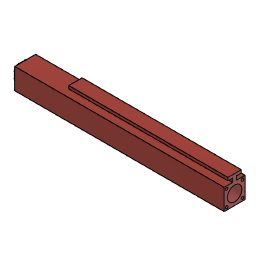
EM2022 Inženýr-ploter (Autodesk Fusion 360 archive; units mm, degrees)
design "EM_22_Plotter_arm_fixa_holder_v7"
Autodesk Fusion 360 part; units mm, degrees
sketch "Sketch7" plane through (0, 0, 0) normal (0, 1, 0) x (1, 0, 0)
sketch "Sketch8" plane through (0, 0, 0) normal (1, 0, 0) x (0, 1, 0)
  circle A0 centre (0, 0) radius 4.6
  line L0 (0, 0) -> (6.5079, 0)
  line L1 (0, 0) -> (0, 4.6)
  line L2 (0, 4.6) -> (0, 6.6)
  line L3 (0, 6.6) -> (6.5777, 6.6)
  line L4 (0, 0) -> (-4.6, 0)
  line L5 (-4.6, 0) -> (-6.6, 0)
  line L6 (0, 0) -> (0, -4.6)
  line L7 (0, -4.6) -> (0, -6.6)
  line L8 (0, -6.6) -> (-6.5261, -6.6)
  line L9 (6.5777, 6.6) -> (-6.5261, 6.6)
  line L10 (-6.5261, -6.6) -> (6.5079, -6.6)
  line L11 (4.6, 0) -> (6.6, 0)
  line L12 (6.6, 0) -> (6.5777, 6.6)
  line L13 (6.5079, 0) -> (6.5079, -6.6)
  line L14 (-6.6, 0) -> (-6.6, -6.5001)
  line L15 (-6.6, 0) -> (-6.6, 6.5001)
  line L16 (0, -6.6) -> (-6.6, -6.6)
  line L17 (-6.6, -6.6) -> (-6.6, -6.4)
  line L18 (-6.5261, 6.6) -> (-6.6, 6.6)
  line L19 (-6.6, 6.6) -> (-6.6, 6.4)
  dimension "d1" = 9.2
  dimension "d2" = 2
  dimension "d3" = 2
  dimension "d4" = 2
  dimension "d5" = 2
  constraint coincident A0.centre L0.start
  constraint horizontal L0
  constraint coincident A0 L1.end
  constraint perpendicular L0 L1
  constraint parallel L1 L2
  constraint perpendicular L2 L3
  constraint coincident A0 L4.end
  constraint perpendicular L1 L4
  constraint parallel L4 L5
  constraint coincident A0 L6.end
  constraint perpendicular L0 L6
  constraint perpendicular L0 L7
  constraint perpendicular L7 L8
  constraint horizontal L9
  constraint horizontal L10
  constraint coincident L0 L11.start
  constraint coincident A0 L11.start
  constraint parallel L0 L11
  constraint perpendicular L10 L13
  constraint vertical L14
  constraint vertical L15
  constraint perpendicular L14 L16
  constraint coincident L14 L17.end
  constraint perpendicular L16 L17
  constraint perpendicular L15 L18
  constraint coincident L15 L19.end
  constraint perpendicular L18 L19
  measures "d1" diameter of A0
  measures "d2" distance of L1.end L2.end
  measures "d3" distance of L4.end L5.end
  measures "d4" distance of L6.end L7.end
  measures "d5" distance of L11.start L11.end
extrude "Extrude1" add sketch "Sketch8" along normal blind 130 contours A0 L0 L7 L10 L11 L13 | A0 L0 L2 L3 L9 L11 L12 | A0 L2 L5 L9 L15 L18 L19 | A0 L5 L7 L8 L10 L14 L16 L17 makes body 1
extrude "Extrude2" add 1 faces at (86.6667, 6.5079, -2.2) along direction (0, 1, 0) blind 0.104 on bodies 1 bodies 1
sketch "Sketch9" plane through (0, 0, 0) normal (-1, 0, 0) x (0, -1, 0)
  circle A0 centre (0, 0) radius 4.6
  line L0 (-6.6, 0) -> (-6.6119, 0)
  line L1 (-6.6119, 0) -> (-6.6119, -6.6)
  line L2 (-6.6119, -6.6) -> (6.6, -6.6)
  line L3 (6.6, -6.6) -> (6.6, 6.6)
  line L4 (6.6, 6.6) -> (-6.5777, 6.6)
  line L5 (-6.5777, 6.6) -> (-6.6, 0)
  circle A1 centre (0, 0) radius 2.75
  line L6 (5, 5) -> (-5, 5)
  line L7 (-5, 5) -> (-5, -5)
  line L8 (-5, -5) -> (5, -5)
  line L9 (5, -5) -> (5, 5)
  dimension "d10" = 5.5
  constraint coincident A0.centre A1.centre
  constraint horizontal L6
  constraint vertical L7
  constraint horizontal L8
  constraint vertical L9
  measures "d10" diameter of A1
extrude "Extrude3" add sketch "Sketch9" along normal blind 4 and the other way blind 0 draft 5 contours A0 | L6 L7 L8 L9 bodies 1
extrude "Extrude4" add 1 faces at (0, 5.5333, 0) along direction (-1, 0, 0) blind 2 on bodies 1 bodies 1
fillet "Fillet1" radius 3 4 edges at (-3, -5, -5) (-3, 5, -5) (-3, -5, 5) (-3, 5, 5) on bodies 1
extrude "Extrude5" cut 1 faces at (42, 6.6119, -4.4) along direction (0, -1, 0) blind 0.002 on bodies 1 bodies 1
fillet "Fillet2" radius 0.6 8 edges at (-4, 4.1213, -4.1213) (-4, 0, -5) (-4, -4.1213, -4.1213) (-4, -5, 0) (-4, -4.1213, 4.1213) (-4, 0, 5) (-4, 4.1213, 4.1213) (-4, 5, 0) on bodies 1
fillet "Fillet3" radius 0.4 8 edges at (-2, -5, 0) (-2, -4.1213, 4.1213) (-2, 0, 5) (-2, 4.1213, 4.1213) (-2, 5, 0) (-2, 4.1213, -4.1213) (-2, 0, -5) (-2, -4.1213, -4.1213) on bodies 1
fillet "Fillet4" radius 0.4 3 edges at (-2, -6.6, 0) (-2, -0.0112, 6.6) (-2, 0.005, -6.6) on bodies 1
sketch "Sketch10" plane through (130, 0, 0) normal (1, 0, 0) x (0, 1, 0)
  line L0 (6.6099, -6.6) -> (6.6099, 0)
  line L1 (6.6099, 0) -> (6.6, 0)
  line L2 (6.6, 0) -> (6.5777, 6.6)
  line L3 (6.5777, 6.6) -> (-6.6, 6.6)
  line L4 (-6.6, 6.6) -> (-6.6, -6.6)
  line L5 (-6.6, -6.6) -> (6.6099, -6.6)
  circle A0 centre (0, 0) radius 4.6
extrude "Extrude6" add sketch "Sketch10" along normal blind 28 separate body makes body 2
sketch "Sketch11" plane through (158, 0, 0) normal (1, 0, 0) x (0, 1, 0)
  circle A0 centre (0, 0) radius 4.6
  line L0 (-6.6, -6.6) -> (6.6099, -6.6)
  line L1 (6.6099, -6.6) -> (6.6099, 0)
  line L2 (6.6099, 0) -> (6.6, 0)
  line L3 (6.6, 0) -> (6.5777, 6.6)
  line L4 (6.5777, 6.6) -> (-6.6, 6.6)
  line L5 (-6.6, 6.6) -> (-6.6, -6.6)
  line L6 (5, 5) -> (-5, 5)
  line L7 (-5, 5) -> (-5, -5)
  line L8 (-5, -5) -> (5, -5)
  line L9 (5, -5) -> (5, 5)
  constraint horizontal L6
  constraint vertical L7
  constraint horizontal L8
  constraint vertical L9
extrude "Extrude7" add sketch "Sketch11" along normal blind 2 and the other way blind 1.5 contours A0 | L6 L7 L8 L9 bodies 2
sketch "Sketch12" plane through (156.5, 0, 0) normal (-1, 0, 0) x (0, -1, 0)
  circle A0 centre (0, 0) radius 4.6
  circle A1 centre (0, 0) radius 2.5
  dimension "d33" = 5
  constraint coincident A0.centre A1.centre
  measures "d33" diameter of A1
extrude "Extrude8" add sketch "Sketch12" along normal blind 26.5 bodies 2
sketch "Sketch13" plane through (130, 0, 0) normal (-1, 0, 0) x (0, -1, 0)
  circle A0 centre (0, 0) radius 2.5
  line L0 (-6.6099, -6.6) -> (6.6, -6.6)
  line L1 (6.6, -6.6) -> (6.6, 6.6)
  line L2 (6.6, 6.6) -> (-6.5777, 6.6)
  line L3 (-6.5777, 6.6) -> (-6.6, 0)
  line L4 (-6.6, 0) -> (-6.6099, 0)
  line L5 (-6.6099, 0) -> (-6.6099, -6.6)
  line L6 (-4, -4) -> (4, -4)
  line L7 (4, -4) -> (4, 4)
  line L8 (4, 4) -> (-4, 4)
  line L9 (-4, 4) -> (-4, -4)
  constraint horizontal L6
  constraint vertical L7
  constraint horizontal L8
  constraint vertical L9
extrude "Extrude9" cut sketch "Sketch13" against normal blind 34 contours L0 L1 L2 L3 L4 L5 bodies 2
sketch "Sketch14" plane through (160, 0, 0) normal (1, 0, 0) x (0, 1, 0)
  line L0 (4, 4) -> (-4, 4)
  line L1 (-4, 4) -> (-4, -4)
  line L2 (-4, -4) -> (4, -4)
  line L3 (4, -4) -> (4, 4)
  line L4 (3, 3) -> (-3, 3)
  line L5 (-3, 3) -> (-3, -3)
  line L6 (-3, -3) -> (3, -3)
  line L7 (3, -3) -> (3, 3)
  constraint horizontal L4
  constraint vertical L5
  constraint horizontal L6
  constraint vertical L7
extrude "Extrude10" add sketch "Sketch14" along normal blind 1 contours L4 L5 L6 L7 bodies 2
sketch "Sketch15" plane through (130, 0, 0) normal (-1, 0, 0) x (0, -1, 0)
  line L0 (4, 4) -> (-4, 4)
  line L1 (-4, 4) -> (-4, -4)
  line L2 (-4, -4) -> (4, -4)
  line L3 (4, -4) -> (4, 4)
  circle A0 centre (0, 0) radius 2.5
  line L4 (5, 5) -> (-5, 5)
  line L5 (-5, 5) -> (-5, -5)
  line L6 (-5, -5) -> (5, -5)
  line L7 (5, -5) -> (5, 5)
  constraint horizontal L4
  constraint vertical L5
  constraint horizontal L6
  constraint vertical L7
extrude "Extrude11" add sketch "Sketch15" against normal blind 30 contours L4 L5 L6 L7 bodies 2
sketch "Sketch16" plane through (130, 0, 0) normal (1, 0, 0) x (0, 1, 0)
  line L0 (6.6099, -6.6) -> (6.6099, 0)
  line L1 (6.6099, 0) -> (6.6, 0)
  line L2 (6.6, 0) -> (6.5777, 6.6)
  line L3 (6.5777, 6.6) -> (-6.6, 6.6)
  line L4 (-6.6, 6.6) -> (-6.6, -6.6)
  line L5 (-6.6, -6.6) -> (6.6099, -6.6)
  circle A0 centre (0, 0) radius 4.6
  circle A1 centre (5, 5) radius 0.85
  circle A2 centre (-5, 5) radius 0.85
  circle A3 centre (5, -5) radius 0.85
  circle A4 centre (-5, -5) radius 0.85
  dimension "d42" = 1.7
  dimension "d43" = 1.7
  dimension "d44" = 1.7
  dimension "d45" = 1.7
  measures "d42" diameter of A1
  measures "d43" diameter of A2
  measures "d44" diameter of A3
  measures "d45" diameter of A4
extrude "Extrude12" cut sketch "Sketch16" against normal blind 7 contours A1 | A2 | A3 | A4 bodies 1
sketch "Sketch17" plane through (160, 0, 0) normal (1, 0, 0) x (0, 1, 0)
  line L0 (-5, 5) -> (-5, -5)
  line L1 (-5, -5) -> (5, -5)
  line L2 (5, -5) -> (5, 5)
  line L3 (5, 5) -> (-5, 5)
  line L4 (3, -3) -> (-3, -3)
  line L5 (-3, -3) -> (-3, 3)
  line L6 (-3, 3) -> (3, 3)
  line L7 (3, 3) -> (3, -3)
  circle A0 centre (5, 5) radius 0.85
  circle A1 centre (-5, 5) radius 0.85
  circle A2 centre (-5, -5) radius 0.85
  circle A3 centre (5, -5) radius 0.85
  circle A4 centre (5, -5) radius 1.6
  circle A5 centre (5, 5) radius 1.6
  circle A6 centre (-5, 5) radius 1.6
  circle A7 centre (-5, -5) radius 1.6
  dimension "d48" = 1.7
  dimension "d49" = 1.7
  dimension "d50" = 1.7
  dimension "d51" = 1.7
  constraint coincident L2.end L3.start
  constraint coincident L0.start L3.end
  constraint coincident L0.end L1.start
  constraint coincident L1.end L2.start
  constraint concentric A3 A4
  constraint concentric A1 A6
  constraint concentric A2 A7
  measures "d48" diameter of A0
  measures "d49" diameter of A1
  measures "d50" diameter of A2
  measures "d51" diameter of A3
extrude "Extrude13" add sketch "Sketch17" along normal blind -30 and the other way blind 27 contours L0 L3 A1 A6 | L0 L1 A2 A7 | L2 L3 A0 A5 | L1 L2 A3 A4 picked at (-6.3454, 4.9461) picked at (-3.6588, -5.1198) picked at (3.9607, 5.8559) picked at (3.656, -5.0795) bodies 2
sketch "Sketch18" plane through (0, 0, 0) normal (0, 0, 1) x (1, 0, 0)
sketch "Sketch19" plane through (130, 0, 0) normal (-1, 0, 0) x (0, -1, 0)
  line L0 (-4.15, 5) -> (-5, 5)
  line L1 (-5, 5) -> (-5, 4.15)
  arc A0 (-4.15, 5) -> (-5, 4.15) centre (-5, 5) ccw
  arc A1 (-3.4, 5) -> (-5, 3.4) centre (-5, 5) ccw
  line L2 (-5, 3.4) -> (-5, -3.4)
  arc A2 (-5, -3.4) -> (-3.4, -5) centre (-5, -5) ccw
  line L3 (-3.4, -5) -> (3.4, -5)
  arc A3 (3.4, -5) -> (5, -3.4) centre (5, -5) ccw
  line L4 (5, -3.4) -> (5, 3.4)
  arc A4 (5, 3.4) -> (3.4, 5) centre (5, 5) ccw
  line L5 (3.4, 5) -> (-3.4, 5)
  line L6 (-5, -4.15) -> (-5, -5)
  line L7 (-5, -5) -> (-4.15, -5)
  arc A5 (-5, -4.15) -> (-4.15, -5) centre (-5, -5) ccw
  arc A6 (4.15, -5) -> (5, -4.15) centre (5, -5) ccw
  line L8 (4.15, -5) -> (5, -5)
  line L9 (5, -5) -> (5, -4.15)
  arc A7 (5, 4.15) -> (4.15, 5) centre (5, 5) ccw
  line L10 (5, 4.15) -> (5, 5)
  line L11 (5, 5) -> (4.15, 5)
  circle A8 centre (0, 0) radius 2.5
  circle A9 centre (-5, 5) radius 0.85
  circle A10 centre (-5, -5) radius 0.85
  circle A11 centre (5, 5) radius 0.85
  circle A12 centre (5, -5) radius 0.85
  constraint coincident L1.end A9
  constraint concentric A2 A10
  constraint coincident L6.start A10
  constraint concentric A4 A11
  constraint concentric A3 A12
extrude "Extrude14" cut sketch "Sketch19" against normal blind 34 contours L0 L1 A9 | L6 L7 A10 | L8 L9 A12 | L10 L11 A11 bodies 2
sketch "Sketch20" plane through (160, 0, 0) normal (1, 0, 0) x (0, 1, 0)
  line L0 (3, -3) -> (-3, -3)
  line L1 (-3, -3) -> (-3, 3)
  line L2 (-3, 3) -> (3, 3)
  line L3 (3, 3) -> (3, -3)
  arc A0 (-5, 4.15) -> (-4.15, 5) centre (-5, 5) ccw
  line L4 (-5, 4.15) -> (-5, -4.15)
  arc A1 (-4.15, -5) -> (-5, -4.15) centre (-5, -5) ccw
  line L5 (-4.15, -5) -> (4.15, -5)
  arc A2 (5, -4.15) -> (4.15, -5) centre (5, -5) ccw
  line L6 (5, -4.15) -> (5, 4.15)
  arc A3 (4.15, 5) -> (5, 4.15) centre (5, 5) ccw
  line L7 (4.15, 5) -> (-4.15, 5)
  circle A4 centre (5, -5) radius 2
  circle A5 centre (5, 5) radius 2
  circle A6 centre (-5, 5) radius 2
  circle A7 centre (-5, -5) radius 2
  line L8 (-5, 5) -> (-5, -5)
  line L9 (-5, -5) -> (5, -5)
  line L10 (5, -5) -> (5, 5)
  line L11 (5, 5) -> (-5, 5)
  dimension "d58" = 4
  dimension "d59" = 4
  dimension "d60" = 4
  dimension "d61" = 4
  constraint concentric A2 A4
  constraint concentric A3 A5
  constraint concentric A0 A6
  constraint concentric A1 A7
  constraint coincident A0.centre A6.centre
  constraint coincident A1.centre A7.centre
  constraint coincident A2.centre A4.centre
  constraint coincident A3.centre A5.centre
  measures "d58" diameter of A4
  measures "d59" diameter of A5
  measures "d60" diameter of A6
  measures "d61" diameter of A7
extrude "Extrude15" cut sketch "Sketch20" against normal blind 27 contours A0 L4 L7 A6 L8 L11 | L4 A1 L5 A7 L8 L9 | L6 A3 L7 A5 L10 L11 | L5 A2 L6 A4 L9 L10 bodies 2
sketch "Sketch21" plane through (130, 0, 0) normal (1, 0, 0) x (0, 1, 0)
  circle A0 centre (-5, -5) radius 0.85
  circle A1 centre (5, 5) radius 0.85
  circle A2 centre (5, -5) radius 0.85
  circle A3 centre (-5, 5) radius 0.85
  line L0 (6.6099, -6.6) -> (6.6099, 0)
  line L1 (6.6099, 0) -> (6.6, 0)
  line L2 (6.6, 0) -> (6.5777, 6.6)
  line L3 (6.5777, 6.6) -> (-6.6, 6.6)
  line L4 (-6.6, 6.6) -> (-6.6, -6.6)
  line L5 (-6.6, -6.6) -> (6.6099, -6.6)
  circle A4 centre (0, 0) radius 4.6
  line L6 (6.5777, 6.6) -> (2.5777, 6.5865)
  line L7 (-0.0112, 6.6) -> (1.1888, 6.6)
  line L8 (2.5777, 6.5865) -> (1.1888, 6.6)
  line L9 (-0.0112, 6.6) -> (-1.2112, 6.6)
  line L10 (-1.2112, 6.6) -> (-1.2112, 9)
  line L11 (1.1888, 6.6) -> (1.1888, 9)
  line L12 (1.1888, 9) -> (4.1888, 9)
  line L13 (-1.2112, 9) -> (-4.2112, 9)
  line L14 (-4.2112, 9) -> (-4.2112, 10.8)
  line L15 (-4.2112, 10.8) -> (5, 10.8)
  line L16 (4.1888, 9) -> (4.1888, 10.8)
  line L17 (-1.2112, 6.6) -> (1.1888, 6.6)
  line L18 (-1.2112, 6.6) -> (-6.6112, 6.6)
  dimension "d73" = 2.4
  dimension "d74" = 3
  dimension "d76" = 1.8
  dimension "d79" = 2.4
  dimension "d81" = 5.4
  constraint coincident L2.end L3.start
  constraint perpendicular L2 L6
  constraint parallel L3 L7
  constraint perpendicular L9 L10
  constraint perpendicular L11 L12
  constraint perpendicular L10 L13
  constraint perpendicular L13 L14
  constraint perpendicular L14 L15
  constraint coincident L15 L16.end
  constraint perpendicular L15 L16
  constraint perpendicular L10 L17
  constraint perpendicular L10 L18
  measures "d73" distance of L7.end L11.end
  measures "d74" distance of L11.end L12.end
  measures "d76" distance of L13.end L14.end
  measures "d79" distance of L9.end L7.end
  measures "d81" distance of L9.end L18.end
extrude "Extrude16" add sketch "Sketch21" against normal blind 100 contours L3 L7 L9 L10 L11 L12 L13 L14 L15 L16 L17 bodies 1
sketch "Sketch22" plane through (0, 0, 0) normal (0, 1, 0) x (1, 0, 0)
sketch "Sketch23" plane through (130, 0, 0) normal (1, 0, 0) x (0, 1, 0)
  circle A0 centre (-5, -5) radius 0.85
  circle A1 centre (5, 5) radius 0.85
  circle A2 centre (5, -5) radius 0.85
  circle A3 centre (-5, 5) radius 0.85
  line L0 (6.6099, -6.6) -> (6.6099, 0)
  line L1 (6.6099, 0) -> (6.6, 0)
  line L2 (6.6, 0) -> (6.5777, 6.6)
  line L3 (6.5777, 6.6) -> (1.1888, 6.6)
  line L4 (1.1888, 6.6) -> (1.1888, 9)
  line L5 (1.1888, 9) -> (4.1888, 9)
  line L6 (4.1888, 9) -> (4.1888, 10.8)
  line L7 (4.1888, 10.8) -> (-4.2112, 10.8)
  line L8 (-4.2112, 10.8) -> (-4.2112, 9)
  line L9 (-4.2112, 9) -> (-1.2112, 9)
  line L10 (-1.2112, 9) -> (-1.2112, 6.6)
  line L11 (-1.2112, 6.6) -> (-6.6, 6.6)
  line L12 (-6.6, 6.6) -> (-6.6, -6.6)
  line L13 (-6.6, -6.6) -> (6.6099, -6.6)
  circle A4 centre (0, 0) radius 4.6
hidden bodies 2
